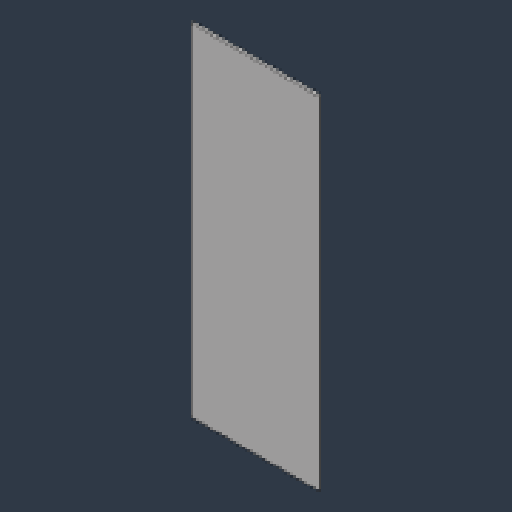
# Autodesk Inventor part: feeder_contact_plate
Saved by Autodesk Inventor 2024.3 (Build 283343000, 343)
## iProperties
Created: 2025-03-07
Part Number: feeder_contact_plate
Material: Generic
Document SubType Name: Sheet Metal
Designer: marcu
Density: 1 g/cm^3
Sheet Metal Rule: Default
Appearance: Default
Author: marcu
Autodesk Inventor part; units mm, degrees
ref_plane "YZ Plane" through (0, 0, 0) normal (1, 0, 0) x (0, 1, 0)
ref_plane "XZ Plane" through (0, 0, 0) normal (0, 1, 0) x (-1, 0, 0)
ref_plane "XY Plane" through (0, 0, 0) normal (0, 0, 1) x (1, 0, 0)
sketch "Sketch1" plane through (0, 0, 0) normal (0, 0, 1) x (1, 0, 0)
  line L0 (76.2, 254) -> (-76.2, 254)
  line L1 (-76.2, 254) -> (-76.2, -254)
  line L2 (-76.2, -254) -> (76.2, -254)
  line L3 (76.2, -254) -> (76.2, 254)
  line L4 (76.2, 254) -> (-76.2, -254) construction
  line L5 (-76.2, 254) -> (76.2, -254) construction
  point P0 (0, 0)
  dimension "d0" = 152.4
  dimension "d1" = 508
  measures "d0" distance of L2.end L1.end
  measures "d1" distance of L1.end L0.end
extrude "Plate1" add sketch "Sketch1" along normal blind 3.048
equation "\"d2\" = Thickness"
equation "\"BendRadius\" = Thickness"
equation "\"BendReliefWidth\" = Thickness"
equation "\"BendReliefDepth\" = 0.5 * Thickness"
equation "\"CornerReliefSize\" = 4 * Thickness"
equation "\"MinimumRemnant\" = 2 * Thickness"
equation "\"TransitionRadius\" = BendRadius"
equation "\"JacobiRadiusSize\" = BendRadius"
equation "\"GapSize\" = Thickness"
equation "\"Thickness\" = 3.048"
body "Solid1"
